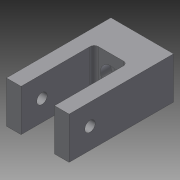
# Autodesk Inventor part: X_Rail_Belt_Pulley_Connector(2)
Saved by Autodesk Inventor 2015 (Build 190159000, 159)
## iProperties
Created: 2017-02-16
Part Number: X_Rail_Belt_Pulley_Connector(2)
Material: Generic
Document SubType Name: Modeling
Designer: Guy
Density: 1 g/cm^3
Appearance: Default
Mass: 17.8501 g
Surface Area: 68.837 cm^2
Volume: 17.8501 cm^3
Author: Guy
Autodesk Inventor part; units mm, degrees
ref_plane "YZ Plane" through (0, 0, 0) normal (1, 0, 0) x (0, 1, 0)
ref_plane "XZ Plane" through (0, 0, 0) normal (0, 1, 0) x (-1, 0, 0)
ref_plane "XY Plane" through (0, 0, 0) normal (0, 0, 1) x (1, 0, 0)
sketch "Sketch1" plane through (0, 0, 0) normal (0, 0, 1) x (1, 0, 0)
  line L0 (0, 0) -> (30, 0)
  line L1 (30, 0) -> (30, 20)
  line L2 (30, 20) -> (0, 20)
  line L3 (0, 20) -> (0, 0)
  dimension "d0" = 30
  dimension "d1" = 20
  constraints: 8 end point, 2 parallel, 1 horizontal, 1 perpendicular
  measures "d0" distance of L2.end L1.end
  measures "d1" distance of L2.end L0.start
extrude "Extrusion1" add sketch "Sketch1" along normal blind 50
sketch "Sketch2" plane through (0, 20, 0) normal (0, 1, 0) x (1, 0, 0)
  line L0 (30, 0) -> (0, 0) projected
  line L1 (0, 0) -> (0, -50) projected
  line L2 (30, -50) -> (0, -50) projected
  line L3 (30, 0) -> (30, -50) projected
  line L4 (7, -50) -> (23, -50)
  line L5 (23, -50) -> (23, -15)
  line L6 (23, -15) -> (7, -15)
  line L7 (7, -15) -> (7, -50)
  point P0 (0, 0)
  dimension "d5" = 7
  dimension "d8" = 15
  dimension "d26" = 7
  constraints: 8 end point, 2 parallel, 1 horizontal, 1 perpendicular, 1 point on line
  measures "d5" distance between parallel lines of L7 L1
  measures "d8" distance between parallel lines of L6 L0
  measures "d26" distance between parallel lines of L3 L5
extrude "Extrusion2" cut sketch "Sketch2" against normal up to next contours L2 L7 L6 L5
sketch "Sketch3" plane through (30, 0, 0) normal (1, 0, 0) x (0, 0, -1)
  line L0 (0, 0) -> (0, 20) projected
  line L1 (0, 20) -> (-50, 20) projected
  line L2 (-50, 0) -> (-50, 20) projected
  line L3 (0, 0) -> (-50, 0) projected
  circle A0 centre (-40, 10) radius 2.5
  point P0 (0, 0)
  dimension "d11" = 5
  dimension "d12" = 10
  dimension "d13" = 10
  constraints: 1 centre point
  measures "d11" diameter of A0
  measures "d12" distance from line of L1 A0.centre
  measures "d13" distance from line of L2 A0.centre
extrude "Extrusion3" cut sketch "Sketch3" against normal through all contours A0
sketch "Sketch4" plane through (7, 20, 15) normal (0, 0, 1) x (1, 0, 0)
  line L0 (16, -20) -> (0, -20) projected
  line L1 (16, 0) -> (16, -20) projected
  line L2 (0, 0) -> (16, 0) projected
  line L3 (0, 0) -> (0, -20) projected
  circle A0 centre (8, -10) radius 5
  line L4 (-7, 0) -> (-7, -20) projected
  dimension "d16" = 10
  dimension "d17" = 10
  dimension "d29" = 15
  constraints: 1 centre point
  measures "d16" diameter of A0
  measures "d17" distance from line of L2 A0.centre
  measures "d29" distance from line of L4 A0.centre
extrude "Extrusion4" cut sketch "Sketch4" against normal blind 5 contours A0
sketch "Sketch5" plane through (15, 10, 10) normal (0, 0, 1) x (1, 0, 0)
  circle A0 centre (0, 0) radius 3.175
  line L0 (8, -10) -> (-8, -10) projected
  line L1 (-8, -10) -> (-8, 10) projected
  line L2 (-15, 10) -> (-15, -10) projected
  dimension "d21" = 6.35
  dimension "d22" = 10
  dimension "d30" = 15
  constraints: 1 centre point
  measures "d21" diameter of A0
  measures "d22" distance from line of L0 A0.centre
  measures "d30" distance from line of L2 A0.centre
extrude "Extrusion5" cut sketch "Sketch5" against normal up to next
fillet "Fillet1" radius 2 1 edges at (7, 10, 15)
fillet "Fillet2" radius 2 1 edges at (23, 10, 15)
body "Solid1"
